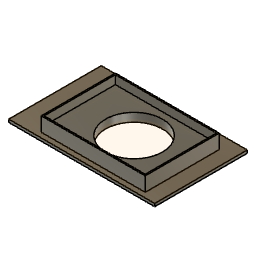
OBS_case_holder (Autodesk Fusion 360 design; units mm, degrees)
Autodesk Fusion 360 part; units mm, degrees
sketch "Sketch1" plane through (0, 0, 0) normal (0, 0, 1) x (1, 0, 0)
  line L0 (0, 0) -> (102.5, 0)
  line L1 (102.5, 0) -> (102.5, 65)
  line L2 (102.5, 65) -> (0, 65)
  line L3 (0, 65) -> (0, 0)
  dimension "d1" = 102.5
  dimension "d2" = 65
  constraint horizontal L0
  constraint vertical L1
  constraint horizontal L2
  constraint vertical L3
  constraint coincident L0.start L3.end
  measures "d1" distance of L0.start L0.end
  measures "d2" distance of L0.start L2.end
extrude "Extrude1" add sketch "Sketch1" along normal blind 2
sketch "Sketch2" plane through (0, 0, 2) normal (0, 0, 1) x (-1, 0, 0)
  line L0 (0, -65) -> (0, 0)
  line L1 (0, 0) -> (-102.5, 0)
  line L2 (-102.5, 0) -> (-102.5, -65)
  line L3 (-102.5, -65) -> (0, -65)
  line L4 (-19.4146, -55.4422) -> (-92.4146, -55.4422)
  line L5 (-92.4146, -55.4422) -> (-92.4146, -3.4422)
  line L6 (-92.4146, -3.4422) -> (-19.4146, -3.4422)
  line L7 (-19.4146, -3.4422) -> (-19.4146, -55.4422)
  dimension "d5" = 73
  dimension "d6" = 52
  constraint horizontal L4
  constraint vertical L5
  constraint horizontal L6
  constraint vertical L7
  measures "d5" distance of L4.start L4.end
  measures "d6" distance of L4.start L6.end
extrude "Extrude2" add sketch "Sketch2" along normal blind 5 contours L4 L5 L6 L7
sketch "Sketch3" plane through (0, 0, 7) normal (0, 0, 1) x (-1, 0, 0)
  line L0 (-19.4146, -3.4422) -> (-92.4146, -3.4422)
  line L1 (-92.4146, -3.4422) -> (-92.4146, -55.4422)
  line L2 (-92.4146, -55.4422) -> (-19.4146, -55.4422)
  line L3 (-19.4146, -55.4422) -> (-19.4146, -3.4422)
  line L4 (-19.4146, -55.4422) -> (-92.4146, -55.4422)
  line L5 (-92.4146, -55.4422) -> (-92.4146, -3.4422)
  line L6 (-92.4146, -3.4422) -> (-19.4146, -3.4422)
  line L7 (-19.4146, -3.4422) -> (-19.4146, -55.4422)
  constraint horizontal L4
  constraint vertical L5
  constraint horizontal L6
  constraint vertical L7
  constraint coincident L0.end L1.start
  constraint coincident L2.end L3.start
extrude "Extrude3" add sketch "Sketch3" along normal blind 5
shell "Shell1" thickness 1 removed faces 1 at (68.0813, 20.7755, 12)
extrude "Extrude4" add 1 faces at (44.0813, 21.1088, 1) along direction (0, 0, 1) blind 5
hole "Hole1" at (57.9907, 30.0204, 6) direction (0, 0, -1) diameter 40 depth 20 tip angle 118
sketch "Sketch4" plane through (0, 0, 2) normal (0, 0, 1) x (-1, 0, 0)
  line L0 (-19.4146, -3.4422) -> (-19.4146, -55.4422)
  line L1 (-19.4146, -55.4422) -> (-92.4146, -55.4422)
  line L2 (-92.4146, -55.4422) -> (-92.4146, -3.4422)
  line L3 (-92.4146, -3.4422) -> (-19.4146, -3.4422)
  line L4 (0, -65) -> (0, 0)
  line L5 (0, 0) -> (-102.5, 0)
  line L6 (-102.5, 0) -> (-102.5, -65)
  line L7 (-102.5, -65) -> (0, -65)
